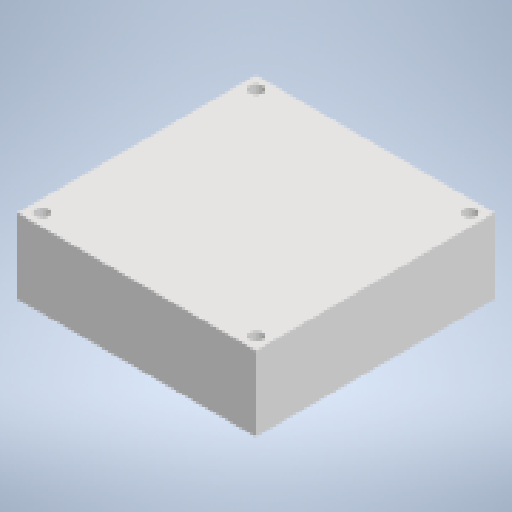
# Autodesk Inventor part: Ventilador
Saved by Autodesk Inventor 2023 (Build 270158000, 158)
## iProperties
Created: 2023-04-03
Part Number: Ventilador
Material: Genérico
Document SubType Name: Modeling
Designer: sergi
Density: 1 g/cm^3
Appearance: Valor por defecto
Author: sergi
Autodesk Inventor part; units mm, degrees
ref_plane "YZ Plane" through (0, 0, 0) normal (1, 0, 0) x (0, 1, 0)
ref_plane "XZ Plane" through (0, 0, 0) normal (0, 1, 0) x (-1, 0, 0)
ref_plane "XY Plane" through (0, 0, 0) normal (0, 0, 1) x (1, 0, 0)
sketch "Boceto1" plane through (0, 0, 0) normal (0, 1, 0) x (-1, 0, 0)
  line L0 (-40, -40) -> (40, -40)
  line L1 (40, -40) -> (40, 40)
  line L2 (40, 40) -> (-40, 40)
  line L3 (-40, 40) -> (-40, -40)
  line L4 (-40, -40) -> (40, 40) construction
  line L5 (40, -40) -> (-40, 40) construction
  point P0 (0, 0)
  dimension "d0" = 80
  dimension "d1" = 80
  constraints: 12 end point, 2 midpoint, 2 parallel, 1 horizontal, 1 perpendicular
  measures "d0" distance of L2.end L1.end
  measures "d1" distance of L1.end L0.end
extrude "Extrusión1" add sketch "Boceto1" along normal blind 25
sketch "Boceto2" plane through (0, 25, 0) normal (0, 1, 0) x (1, 0, 0)
  line L0 (-40, -40) -> (40, -40) projected
  line L1 (40, -40) -> (40, 40) projected
  circle A0 centre (35.8, -35.8) radius 2.1
  line L2 (40, 40) -> (35.8, 40)
  line L3 (40, 40) -> (-40, 40) projected
  line L4 (35.8, 40) -> (40, 40)
  line L5 (-40, 40) -> (-40, -40) projected
  line L6 (-40, 40) -> (-35.8, 40)
  line L7 (-35.8, 40) -> (-35.8, 35.8)
  line L8 (-40, -40) -> (-35.8, -40)
  line L9 (-35.8, -40) -> (-35.8, -35.8)
  circle A1 centre (-35.8, -35.8) radius 2.1
  circle A2 centre (-35.8, 35.8) radius 2.1
  line L10 (35.8, 40) -> (35.8, 35.8)
  circle A3 centre (35.8, 35.8) radius 2.1
  point P0 (0, 0)
  dimension "d15" = 4.2
  dimension "d16" = 4.2
  dimension "d17" = 4.2
  dimension "d18" = 4.2
  dimension "d19" = 4.2
  dimension "d20" = 4.2
  dimension "d21" = 4.2
  dimension "d22" = 4.2
  dimension "d23" = 4.2
  dimension "d24" = 4.2
  constraints: 14 end point, 4 centre point, 3 coincident, 3 perpendicular, 3 point on line, 1 collinear
  measures "d15" distance of L1.end L2.end
  measures "d16" distance of L2.end L1.end
  measures "d17" distance of L3.end L6.end
  measures "d18" distance of L6.end L7.end
  measures "d19" distance of L0.start L8.end
  measures "d20" distance of L8.end L9.end
  measures "d21" diameter of A1
  measures "d22" diameter of A2
  measures "d23" distance of L2.end L10.end
  measures "d24" diameter of A3
hole "Agujero1" at (35.8, 25, 35.8) at (35.8, 25, -35.8) at (-35.8, 25, -35.8) at (-35.8, 25, 35.8) direction (0, -1, 0) diameter 4.25 depth 30
